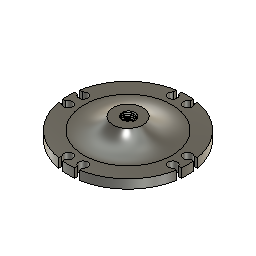
F-machine platten tie down v1.b v1 (Autodesk Fusion 360 design; units mm, degrees)
Autodesk Fusion 360 part; units mm, degrees
sketch "Sketch1" plane through (0, 0, 0) normal (0, 0, 1) x (1, 0, 0)
  circle A0 centre (0, 0) radius 40
  circle A1 centre (-35, -5) radius 3
  circle A2 centre (-35, 5) radius 3
  line L0 (0, 51) -> (0, -22) construction
  circle A3 centre (5, 35) radius 3
  circle A4 centre (35, 5) radius 3
  circle A5 centre (-5, 35) radius 3
  circle A6 centre (-5, -35) radius 3
  circle A7 centre (5, -35) radius 3
  circle A8 centre (35, -5) radius 3
  dimension "d1" = 80
  dimension "d2" = 6
  dimension "d3" = 6
  dimension "d4" = 6
  dimension "d5" = 6
  constraint coincident A0.centre origin
  constraint vertical L0
  constraint symmetric A2 L0 A4
  measures "d1" diameter of A0
  measures "d2" diameter of A1
  measures "d3" diameter of A2
  measures "d4" diameter of A7
  measures "d5" diameter of A6
extrude "Extrude1" add sketch "Sketch1" along normal blind 6
sketch "Sketch2" plane through (0, 0, 6) normal (0, 0, 1) x (-1, 0, 0)
  circle A0 centre (5, -35) radius 3
  circle A1 centre (35, 5) radius 3
  circle A2 centre (-5, -35) radius 3
  circle A3 centre (35, -5) radius 3
  circle A4 centre (-35, -5) radius 3
  circle A5 centre (-5, 35) radius 3
  circle A6 centre (5, 35) radius 3
  circle A7 centre (-35, 5) radius 3
  circle A8 centre (0, 0) radius 40
  circle A9 centre (0, 0) radius 10
  dimension "d8" = 20
  constraint coincident A8.centre A9.centre
  measures "d8" diameter of A9
extrude "Extrude2" add sketch "Sketch2" along normal blind 8 contours A9
fillet "Fillet1" radius 27.5 1 edges at (9.3233, -3.6162, 6)
sketch "Sketch3" plane through (0, 0, 6) normal (0, 0, 1) x (-1, 0, 0)
  circle A0 centre (0, 0) radius 40
  circle A1 centre (-35, 5) radius 3
  circle A2 centre (5, 35) radius 3
  circle A3 centre (-5, 35) radius 3
  circle A4 centre (-35, -5) radius 3
  circle A5 centre (35, -5) radius 3
  circle A6 centre (-5, -35) radius 3
  circle A7 centre (35, 5) radius 3
  circle A8 centre (5, -35) radius 3
  circle A9 centre (0, 0) radius 29.3907
  line L0 (-35, -5) -> (-45.5326, -5) construction
  line L1 (-35, 5) -> (-44, 5) construction
  line L2 (-35, 7) -> (-44, 7)
  line L3 (-35, 4) -> (-44, 4)
  line L4 (-35, -4) -> (-45.5326, -4)
  line L5 (-35, -7) -> (-45.5326, -7)
  line L6 (5, -35) -> (5, -45.5326) construction
  line L7 (7, -35) -> (7, -45.5326)
  line L8 (4, -35) -> (4, -45.5326)
  line L9 (-7, -35) -> (-7, -44)
  line L10 (-5, -35) -> (-5, -44) construction
  line L11 (-4, -35) -> (-4, -44)
  line L12 (35, 5) -> (45.5326, 5) construction
  line L13 (35, -7) -> (44, -7)
  line L14 (35, 4) -> (45.5326, 4)
  line L15 (35, -4) -> (44, -4)
  line L16 (35, -5) -> (44, -5) construction
  line L17 (35, 7) -> (45.5326, 7)
  line L18 (-4, 35) -> (-4, 45.5326)
  line L19 (4, 35) -> (4, 44)
  line L20 (-5, 35) -> (-5, 45.5326) construction
  line L21 (-7, 35) -> (-7, 45.5326)
  line L22 (5, 35) -> (5, 44) construction
  line L23 (7, 35) -> (7, 44)
  dimension "d13" = 2
  dimension "d14" = -1
  dimension "d15" = 1
  dimension "d16" = -2
  dimension "d17" = 2
  dimension "d18" = -1
  dimension "d19" = 1
  dimension "d20" = -2
  dimension "d21" = 2
  dimension "d22" = -1
  dimension "d23" = 1
  dimension "d24" = -2
  constraint coincident A4.centre L0.start
  constraint horizontal L0
  constraint coincident A1.centre L1.start
  constraint horizontal L1
  constraint parallel L6 L8
  constraint parallel L6 L7
  constraint parallel L9 L10
  constraint parallel L10 L11
  constraint parallel L18 L20
  constraint parallel L20 L21
  constraint parallel L22 L23
  constraint parallel L19 L22
  constraint parallel L12 L14
  constraint parallel L12 L17
  constraint parallel L13 L16
  constraint parallel L15 L16
extrude "Extrude3" cut sketch "Sketch3" against normal blind 12 contours A0 A7 L14 L17 | A0 A5 L13 L15 | A0 A2 L19 L23 | A0 A8 L7 L8 | A0 A3 L18 L21 | A0 A6 L9 L11 | A0 A1 L2 L3 | A0 A4 L4 L5
sketch "Sketch4" plane through (0, 0, 14) normal (0, 0, 1) x (-1, 0, 0)
  circle A0 centre (0, 0) radius 10
  circle A1 centre (0, 0) radius 4.7625
  dimension "d27" = 9.525
  constraint concentric A0 A1
  measures "d27" diameter of A1
extrude "Extrude4" cut sketch "Sketch4" against normal blind 12 contours A1
thread "Thread1" "ISO Metric profile 9.0 M9x1.25 6H" major diameter 9.1702 minor diameter 7.7793 pitch 1.25 angle 60 modelled right hand crest width 0.3428 on face at (-4.7566, 0.2374, 6) crest through (-3.8897, 0, 13.6875)
sketch "Sketch5" plane through (0, 0, 0) normal (0, 0, -1) x (1, 0, 0)
  circle A0 centre (0, 0) radius 3.1
  line L0 (37.2361, 7) -> (39.3827, 7)
  arc A1 (39.3827, 7) -> (7, 39.3827) centre (0, 0) ccw
  line L1 (7, 39.3827) -> (7, 37.2361)
  arc A2 (4, 37.8284) -> (7, 37.2361) centre (5, 35) ccw
  line L2 (4, 37.8284) -> (4, 39.7995)
  arc A3 (4, 39.7995) -> (-4, 39.7995) centre (0, 0) ccw
  line L3 (-4, 39.7995) -> (-4, 37.8284)
  arc A4 (-7, 37.2361) -> (-4, 37.8284) centre (-5, 35) ccw
  line L4 (-7, 37.2361) -> (-7, 39.3827)
  arc A5 (-7, 39.3827) -> (-39.3827, 7) centre (0, 0) ccw
  line L5 (-39.3827, 7) -> (-37.2361, 7)
  arc A6 (-37.8284, 4) -> (-37.2361, 7) centre (-35, 5) ccw
  line L6 (-37.8284, 4) -> (-39.7995, 4)
  arc A7 (-39.7995, 4) -> (-39.7995, -4) centre (0, 0) ccw
  line L7 (-39.7995, -4) -> (-37.8284, -4)
  arc A8 (-37.2361, -7) -> (-37.8284, -4) centre (-35, -5) ccw
  line L8 (-37.2361, -7) -> (-39.3827, -7)
  arc A9 (-39.3827, -7) -> (-7, -39.3827) centre (0, 0) ccw
  line L9 (-7, -39.3827) -> (-7, -37.2361)
  arc A10 (-4, -37.8284) -> (-7, -37.2361) centre (-5, -35) ccw
  line L10 (-4, -37.8284) -> (-4, -39.7995)
  arc A11 (-4, -39.7995) -> (4, -39.7995) centre (0, 0) ccw
  line L11 (4, -39.7995) -> (4, -37.8284)
  arc A12 (7, -37.2361) -> (4, -37.8284) centre (5, -35) ccw
  line L12 (7, -37.2361) -> (7, -39.3827)
  arc A13 (7, -39.3827) -> (39.3827, -7) centre (0, 0) ccw
  line L13 (39.3827, -7) -> (37.2361, -7)
  arc A14 (37.8284, -4) -> (37.2361, -7) centre (35, -5) ccw
  line L14 (37.8284, -4) -> (39.7995, -4)
  arc A15 (39.7995, -4) -> (39.7995, 4) centre (0, 0) ccw
  line L15 (39.7995, 4) -> (37.8284, 4)
  arc A16 (37.2361, 7) -> (37.8284, 4) centre (35, 5) ccw
  circle A17 centre (0, 0) radius 5
  dimension "d30" = 10
  constraint concentric A0 A17
  measures "d30" diameter of A17
extrude "Extrude5" [rolled back] along distance -8 taper angle 0
